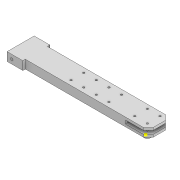
# Autodesk Inventor part: RobotBaseMotorExt
Saved by Autodesk Inventor 2022 (Build 260153000, 153)
## iProperties
Created: 2022-10-20
Part Number: RobotBaseMotorExt
Material: Generic
Document SubType Name: Modeling
Designer: MVeszpremi
Density: 1 g/cm^3
Appearance: Default
Author: MVeszpremi
Autodesk Inventor part; units mm, degrees
sketch "Sketch1" plane through (0, 0, 0) normal (0, 1, 0) x (-1, 0, 0)
  line L0 (0, 0) -> (220, 0)
  line L1 (220, 0) -> (220, -43)
  line L2 (220, -43) -> (0, -43)
  line L3 (0, -43) -> (0, 0)
  line L4 (10, -12.5) -> (30, -12.5)
  line L5 (30, -12.5) -> (30, -32.5)
  line L6 (30, -32.5) -> (10, -32.5)
  line L7 (10, -32.5) -> (10, -12.5)
  circle A0 centre (10, -12.5) radius 1.5
  circle A1 centre (30, -32.5) radius 1.5
  circle A2 centre (30, -12.5) radius 1.5
  circle A3 centre (10, -32.5) radius 1.5
  line L8 (220, 0) -> (195, 0)
  line L9 (195, 0) -> (195, -43)
  line L10 (195, -43) -> (220, -43)
  line L11 (220, -43) -> (220, 0)
  line L12 (195, -4) -> (0, -4)
  line L13 (0, -4) -> (0, -39)
  line L14 (0, -39) -> (195, -39)
  line L15 (195, -39) -> (195, -4)
  line L16 (36, -4) -> (36, -39)
  point P0 (195, 0)
  point P1 (0, -4)
  dimension "d0" = 220
  dimension "d1" = 43
  dimension "d2" = 20
  dimension "d3" = 20
  dimension "d4" = 12.5
  dimension "d5" = 10
  dimension "d6" = 3
  dimension "d7" = 3
  dimension "d8" = 3
  dimension "d9" = 3
  dimension "d18" = 4
  dimension "d19" = 4
  dimension "d23" = 36
  dimension "d66" = 25
  constraints: 34 end point, 8 parallel, 5 perpendicular, 5 point on line, 4 centre point, 4 coincident, 4 horizontal
  measures "d0" distance of L1.end L2.end
  measures "d1" distance of L0.end L1.end
  measures "d2" distance of L4.start L4.end
  measures "d3" distance of L4.end L5.end
  measures "d4" distance between parallel lines of L0 L4
  measures "d5" distance between parallel lines of L3 L7
  measures "d6" diameter of A2
  measures "d7" diameter of A1
  measures "d8" diameter of A3
  measures "d9" diameter of A0
  measures "d18" distance between parallel lines of L0 L12
  measures "d19" distance between parallel lines of L2 L14
  measures "d23" distance between parallel lines of L13 L16
  measures "d66" distance between parallel lines of L1 L9
extrude "Extrusion1" add sketch "Sketch1" along normal blind 4 contours L0 L1 L2 L9 | L12 L16 L14 L3 | L9 L14 L16 L12 | L4 A2 L5 A1 L6 A3 L7 A0
extrude "Extrusion2" add sketch "Sketch1" against normal blind 5.5 contours L0 L1 L2 L9 | L9 L14 L16 L12
ref_plane "Work Plane1" through (0, -2.75, 0) normal (0, -1, 0) x (1, 0, 0)
mirror "Mirror1" about plane through (0, -2.75, 0) normal (0, -1, 0) of "Extrusion1"
chamfer "Chamfer1" distance 7.5 angle 45 4 edges at (0, 2, -4) (0, -7.5, -4) (0, -7.5, -39) (0, 2, -39)
ref_plane "Work Plane2" through (-152.5, -8.5, -20) normal (0, 0, -1) x (-1, 0, 0)
sketch "Sketch5" plane through (-195, -9.5, -39) normal (0, -1, 0) x (1, 0, 0)
  circle A0 centre (165, 26.5) radius 1.5 projected
  line L0 (165, 29.9641) -> (168, 28.2321)
  line L1 (168, 28.2321) -> (168, 24.7679)
  line L2 (168, 24.7679) -> (165, 23.0359)
  line L3 (165, 23.0359) -> (162, 24.7679)
  line L4 (162, 24.7679) -> (162, 28.2321)
  line L5 (162, 28.2321) -> (165, 29.9641)
  circle A1 centre (185, 26.5) radius 1.5 projected
  line L6 (185, 29.9641) -> (188, 28.2321)
  line L7 (188, 28.2321) -> (188, 24.7679)
  line L8 (188, 24.7679) -> (185, 23.0359)
  line L9 (185, 23.0359) -> (182, 24.7679)
  line L10 (182, 24.7679) -> (182, 28.2321)
  line L11 (182, 28.2321) -> (185, 29.9641)
  circle A2 centre (185, 6.5) radius 1.5 projected
  line L12 (185, 9.9641) -> (188, 8.2321)
  line L13 (188, 8.2321) -> (188, 4.7679)
  line L14 (188, 4.7679) -> (185, 3.0359)
  line L15 (185, 3.0359) -> (182, 4.7679)
  line L16 (182, 4.7679) -> (182, 8.2321)
  line L17 (182, 8.2321) -> (185, 9.9641)
  circle A3 centre (165, 6.5) radius 1.5 projected
  line L18 (165, 9.9641) -> (168, 8.2321)
  line L19 (168, 8.2321) -> (168, 4.7679)
  line L20 (168, 4.7679) -> (165, 3.0359)
  line L21 (165, 3.0359) -> (162, 4.7679)
  line L22 (162, 4.7679) -> (162, 8.2321)
  line L23 (162, 8.2321) -> (165, 9.9641)
  circle A4 centre (165, 26.5) radius 5.25
  circle A5 centre (185, 26.5) radius 5.25
  circle A6 centre (185, 6.5) radius 5.25
  circle A7 centre (165, 6.5) radius 5.25
  point P0 (195, 39)
  dimension "d44" = 6
  dimension "d45" = 6
  dimension "d46" = 6
  dimension "d47" = 6
  dimension "d48" = 10.5
  dimension "d49" = 10.5
  dimension "d50" = 10.5
  dimension "d51" = 10.5
  constraints: 48 end point, 8 coincident, 4 centre point, 52 other
  measures "d44" distance between parallel lines of L1 L4
  measures "d45" distance between parallel lines of L7 L10
  measures "d46" distance between parallel lines of L13 L16
  measures "d47" distance between parallel lines of L19 L22
  measures "d48" diameter of A4
  measures "d49" diameter of A5
  measures "d50" diameter of A7
  measures "d51" diameter of A6
extrude "Extrusion5" add sketch "Sketch5" along normal blind 3.5 contours A4 | A5 | A6 | A7
sketch "Sketch6" plane through (-195, -9.5, -39) normal (0, -1, 0) x (1, 0, 0)
  circle A0 centre (65, 7.5) radius 1.5
  line L0 (187.5, 0) -> (0, 0) projected
  line L1 (0, 0) -> (0, -4) projected
  circle A1 centre (85, 7.5) radius 1.5
  circle A2 centre (105, 7.5) radius 1.5
  circle A3 centre (125, 7.5) radius 1.5
  point P0 (195, 39)
  point P1 (0, -5)
  dimension "d54" = 3
  dimension "d55" = 7.5
  dimension "d56" = 65
  dimension "d59" = 20
  constraints: 4 centre point, 1 horizontal, 6 other
  measures "d54" diameter of A0
  measures "d55" distance from line of L0 A0.centre
  measures "d56" distance from line of L1 A0.centre
  measures "d59" distance of A0.centre A1.centre
extrude "Extrusion6" cut sketch "Sketch6" against normal blind 33.25
ref_plane "Work Plane3" through (-195, -9.5, -21.5) normal (0, 0, -1) x (-1, 0, 0)
mirror "Mirror2" about plane through (-195, -9.5, -21.5) normal (0, 0, -1) of "Extrusion6"
sketch "Sketch7" plane through (-220, 4, 0) normal (0, 0, 1) x (1, 0, 0)
  point P0 (220, -4)
ref_plane "Work Plane4" through (-195, -9.5, -21.5) normal (0, 0, 1) x (1, 0, 0)
sketch "Sketch9" plane through (-220, 4, 0) normal (0, 0, 1) x (1, 0, 0)
  circle A0 centre (7.5, -6.75) radius 2
  line L0 (0, -13.5) -> (0, 0) projected
  line L1 (0, 0) -> (25, 0) projected
  point P0 (220, -4)
  dimension "d75" = 4
  dimension "d76" = 7.5
  dimension "d77" = 6.75
  constraints: 1 centre point
  measures "d75" diameter of A0
  measures "d76" distance from line of L0 A0.centre
  measures "d77" distance from line of L1 A0.centre
extrude "Extrusion8" cut sketch "Sketch9" against normal blind 73.25
body "Solid1"
